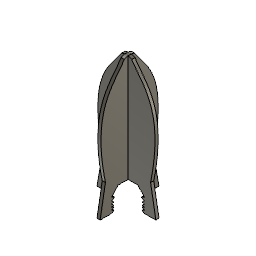
NYE-Rocket (Autodesk Fusion 360 design; units mm, degrees)
part number: 2025-12-20-13-37-46-259
Autodesk Fusion 360 part; units mm, degrees
sketch "Sketch1" plane through (0, 0, 0) normal (0, 1, 0) x (1, 0, 0)
  arc A0 (-14.7, 0) -> (-13.8108, -14.2595) centre (8.3307, -5.7213) ccw construction
  line L0 (0, 0) -> (0, -143.1953)
  line L1 (-11.7114, -15.7) -> (-12.05, -15.7) construction
  line L2 (-10.3, -17.45) -> (-10.3, -17.2374) construction
  arc A1 (-13.8108, -14.2595) -> (-11.7114, -15.7) centre (-11.7114, -13.45) ccw construction
  arc A2 (-10.3, -17.45) -> (-12.05, -15.7) centre (-12.05, -17.45) ccw construction
  arc A3 (-10.3, -17.2374) -> (-9.3791, -18.4433) centre (-9.05, -17.2374) ccw construction
  line L3 (11.7114, -15.7) -> (12.05, -15.7) construction
  arc A4 (11.7114, -15.7) -> (13.8108, -14.2595) centre (11.7114, -13.45) ccw construction
  arc A5 (13.8108, -14.2595) -> (14.7, 0) centre (-8.3307, -5.7213) ccw construction
  arc A6 (12.05, -15.7) -> (10.3, -17.45) centre (12.05, -17.45) ccw construction
  arc A7 (9.3791, -18.4433) -> (10.3, -17.2374) centre (9.05, -17.2374) ccw construction
  line L4 (10.3, -17.45) -> (10.3, -17.2374) construction
  arc A8 (0, -19.7) -> (9.3791, -18.4433) centre (0, 15.9286) ccw construction
  line L5 (-14.7, 0) -> (14.7, 0) construction
  line L6 (-27.5, 0) -> (-22.5628, -28)
  arc A9 (-5, -118.6603) -> (5, -118.6603) centre (0, -110) ccw
  line L7 (-22.5628, -28) -> (-35.5651, -92.1831) construction
  line L8 (-35.5651, -92.1831) -> (-14.6245, -102.766) construction
  line L9 (-14.6245, -102.766) -> (-5, -118.6603) construction
  spline S0 degree 3 poles (-22.5628, -28) (-35.5651, -92.1831) (-14.6245, -102.766) (-5, -118.6603) knots 0 0 0 0 1 1 1 1
  line L10 (-27.5, 0) -> (-16.6335, 0)
  line L11 (-16.6335, 0) -> (-14.2715, -1.5)
  line L12 (-14.2715, -1.5) -> (-16.6335, -2.7339)
  line L13 (-16.6335, -2.7339) -> (-14.6044, -4.2507)
  line L14 (-14.6044, -4.2507) -> (-16.6335, -5.1213)
  line L15 (-16.6335, -5.1213) -> (-14.65, -5.7122)
  line L16 (-14.65, -5.7122) -> (-16.6335, -7.5886)
  line L17 (-16.6335, -7.5886) -> (-14.5182, -8.2188)
  line L18 (-14.5182, -8.2188) -> (-16.6335, -10.2198)
  line L19 (-16.6335, -10.2198) -> (-13.8558, -11.8091)
  line L20 (-13.8558, -11.8091) -> (-16.6335, -13.4273)
  line L21 (-16.6335, -13.4273) -> (-10.5442, -19.9101)
  line L22 (-10.5442, -19.9101) -> (0, -19.9101)
  spline S1 degree 3 poles (22.5628, -28) (35.5651, -92.1831) (14.6245, -102.766) (5, -118.6603) knots 0 0 0 0 1 1 1 1
  line L23 (22.5628, -28) -> (35.5651, -92.1831) construction
  line L24 (35.5651, -92.1831) -> (14.6245, -102.766) construction
  line L25 (14.6245, -102.766) -> (5, -118.6603) construction
  line L26 (27.5, 0) -> (22.5628, -28)
  line L27 (27.5, 0) -> (16.6335, 0)
  line L28 (16.6335, -5.1213) -> (14.65, -5.7122)
  line L29 (14.65, -5.7122) -> (16.6335, -7.5886)
  line L30 (16.6335, -7.5886) -> (14.5182, -8.2188)
  line L31 (14.5182, -8.2188) -> (16.6335, -10.2198)
  line L32 (16.6335, -10.2198) -> (13.8558, -11.8091)
  line L33 (13.8558, -11.8091) -> (16.6335, -13.4273)
  line L34 (16.6335, -13.4273) -> (10.5442, -19.9101)
  line L35 (10.5442, -19.9101) -> (0, -19.9101)
  line L36 (14.6044, -4.2507) -> (16.6335, -5.1213)
  line L37 (16.6335, 0) -> (14.2715, -1.5)
  line L38 (14.2715, -1.5) -> (16.6335, -2.7339)
  line L39 (16.6335, -2.7339) -> (14.6044, -4.2507)
  line L40 (-1.575, -119.8752) -> (-1.575, -69.8752)
  line L41 (-1.575, -69.8752) -> (0, -69.8752)
  line L42 (1.575, -69.8752) -> (0, -69.8752)
  line L43 (1.575, -119.8752) -> (1.575, -69.8752)
  point P0 (-13.2, -15.7)
  point P1 (-10.3, -15.7)
  point P2 (10.3, -15.7)
  point P3 (13.2, -15.7)
  point P4 (-15.0215, -1.5)
  point P5 (-15.3544, -4.2507)
  point P6 (-15.4, -5.7122)
  point P7 (-15.2682, -8.2188)
  point P8 (-14.6058, -11.8091)
  dimension "d1" = 26.4
  dimension "d3" = 29.4
  dimension "d4" = 20.6
  dimension "d5" = 2.25
  dimension "d6" = 1.75
  dimension "d8" = 15.7
  dimension "d9" = 15.4
  dimension "d10" = 1.25
  dimension "d13" = 120
  dimension "d15" = 55
  dimension "d16" = 10
  dimension "d17" = 10
  dimension "d19" = 28
  dimension "d20" = 80
  dimension "d22" = 60
  dimension "d23" = 60
  dimension "d25" = 0.75
  dimension "d26" = 0.75
  dimension "d27" = 0.75
  dimension "d28" = 0.75
  dimension "d30" = 60
  dimension "d31" = 60
  dimension "d32" = 60
  dimension "d33" = 0.75
  dimension "d34" = 1.5
  dimension "d35" = 3.15
  dimension "d37" = 50
  constraint coincident L0.start origin
  constraint vertical L0
  constraint horizontal L1
  constraint perpendicular L1 L2
  constraint coincident P0 L1
  constraint coincident P0 A0
  constraint tangent A0 A1
  constraint tangent L1 A1
  constraint coincident P1 L1
  constraint coincident P1 L2
  constraint tangent L1 A2
  constraint tangent L2 A2
  constraint horizontal L0.start A0.start
  constraint tangent L2 A3
  constraint symmetric P0 L0 P3
  constraint symmetric A0.start L0 A5.end
  constraint symmetric A0 L0 A5
  constraint symmetric L0 P1 P2
  constraint symmetric L0 L1.start L3.start
  constraint symmetric L0 A0.end A4.end
  constraint symmetric L0 A1 A4
  constraint symmetric L0 L1.end L3.end
  constraint symmetric L0 L2.start A6.end
  constraint symmetric L0 A2 A6
  constraint symmetric L0 L2.end A7.end
  constraint symmetric L0 A3.end A7.start
  constraint symmetric L0 A3 A7
  constraint coincident A0.start L5.start
  constraint coincident A5.end L5.end
  constraint horizontal L0.start L6.start
  constraint symmetric L0 A9.start A9.end
  constraint parallel L5 L10
  constraint parallel L15 L17
  constraint coincident L0 L22.end
  constraint perpendicular L0 L22
  constraint coincident A0 P4
  constraint horizontal L11.end P4
  constraint coincident A0 P5
  constraint horizontal L13.end P5
  constraint coincident A0 P6
  constraint horizontal L15.end P6
  constraint coincident A0 P7
  constraint horizontal L17.end P7
  constraint coincident A0 P8
  constraint horizontal L19.end P8
  constraint vertical L18.end L20.end
  constraint vertical L16.end L18.end
  constraint vertical L14.end L16.end
  constraint vertical L12.end L14.end
  constraint vertical L10.end L12.end
  constraint symmetric L0 L6.start L26.start
  constraint symmetric L0 L6.end S1.start
  constraint symmetric L0 S0 S1
  constraint symmetric L0 L10.end L27.end
  constraint symmetric L0 L11.end L37.end
  constraint symmetric L0 L12.end L38.end
  constraint symmetric L0 L13.end L36.start
  constraint symmetric L0 L14.end L28.start
  constraint symmetric L0 L15.end L28.end
  constraint symmetric L0 L16.end L29.end
  constraint symmetric L0 L17.end L30.end
  constraint symmetric L0 L18.end L31.end
  constraint symmetric L0 L19.end L32.end
  constraint symmetric L0 L20.end L33.end
  constraint symmetric L0 L21.end L34.end
  constraint symmetric L0 L22.end L35.end
  constraint coincident A9 L40.start
  constraint vertical L40
  constraint perpendicular L40 L41
  constraint symmetric L0 L40.start L43.start
  constraint symmetric L0 L40.end L42.start
  constraint symmetric L0 L41.end L42.end
  measures "d5" radius of A1
  measures "d6" radius of A2
  measures "d8" vertical distance of A0.start L1.start
  measures "d9" distance of A0 L0
  measures "d10" radius of A3
  measures "d16" distance of A9.start A9.end
  measures "d17" radius of A9
  measures "d19" vertical distance of L6.start L6.end
  measures "d20" angle of L5 L6
  measures "d22" angle of L11 L12
  measures "d23" angle of L13 L14
  measures "d25" distance of L11.end P4
  measures "d26" distance of L13.end P5
  measures "d27" distance of L15.end P6
  measures "d28" distance of L17.end P7
  measures "d30" angle of L15 L16
  measures "d31" angle of L17 L18
  measures "d32" angle of L19 L20
  measures "d33" distance of L19.end P8
  measures "d34" distance of L10 L11.end
  measures "d37" distance of L40.start L40.end
sketch "Sketch3" plane through (0, 0, 0) normal (1, 0, 0) x (0, 1, 0)
  line L0 (1.575, -119.8752) -> (1.575, -69.8752)
  arc A0 (-10.3, -17.2374) -> (-9.3791, -18.4433) centre (-9.05, -17.2374) ccw construction
  line L1 (-16.6335, -5.1213) -> (-14.65, -5.7122)
  line L2 (-14.7, 0) -> (14.7, 0) construction
  line L3 (-16.6335, -2.7339) -> (-14.6044, -4.2507)
  line L4 (-10.3, -17.45) -> (-10.3, -17.2374) construction
  line L5 (1.575, -69.8752) -> (0, -69.8752)
  spline S0 degree 3 poles (-22.5628, -28) (-35.5651, -92.1831) (-14.6245, -102.766) (-5, -118.6603) knots 0 0 0 0 1 1 1 1
  line L6 (-22.5628, -28) -> (-35.5651, -92.1831) construction
  line L7 (-35.5651, -92.1831) -> (-14.6245, -102.766) construction
  line L8 (-14.6245, -102.766) -> (-5, -118.6603) construction
  line L9 (-10.5442, -19.9101) -> (0, -19.9101)
  line L10 (-16.6335, 0) -> (-14.2715, -1.5)
  line L11 (-27.5, 0) -> (-22.5628, -28)
  arc A1 (-14.7, 0) -> (-13.8108, -14.2595) centre (8.3307, -5.7213) ccw construction
  line L12 (27.5, 0) -> (22.5628, -28)
  arc A2 (-10.3, -17.45) -> (-12.05, -15.7) centre (-12.05, -17.45) ccw construction
  spline S1 degree 3 poles (22.5628, -28) (35.5651, -92.1831) (14.6245, -102.766) (5, -118.6603) knots 0 0 0 0 1 1 1 1
  line L13 (22.5628, -28) -> (35.5651, -92.1831) construction
  line L14 (35.5651, -92.1831) -> (14.6245, -102.766) construction
  line L15 (14.6245, -102.766) -> (5, -118.6603) construction
  line L16 (-1.575, -69.8752) -> (0, -69.8752)
  line L17 (-1.575, -119.8752) -> (-1.575, -69.8752)
  line L18 (16.6335, 0) -> (14.2715, -1.5)
  line L19 (14.6044, -4.2507) -> (16.6335, -5.1213)
  line L20 (14.2715, -1.5) -> (16.6335, -2.7339)
  line L21 (16.6335, -7.5886) -> (14.5182, -8.2188)
  line L22 (14.5182, -8.2188) -> (16.6335, -10.2198)
  line L23 (-16.6335, -7.5886) -> (-14.5182, -8.2188)
  line L24 (-14.5182, -8.2188) -> (-16.6335, -10.2198)
  line L25 (14.65, -5.7122) -> (16.6335, -7.5886)
  line L26 (-16.6335, -10.2198) -> (-13.8558, -11.8091)
  line L27 (-16.6335, -13.4273) -> (-10.5442, -19.9101)
  line L28 (-14.2715, -1.5) -> (-16.6335, -2.7339)
  line L29 (-11.7114, -15.7) -> (-12.05, -15.7) construction
  arc A3 (-13.8108, -14.2595) -> (-11.7114, -15.7) centre (-11.7114, -13.45) ccw construction
  line L30 (-27.5, 0) -> (-16.6335, 0)
  arc A4 (9.3791, -18.4433) -> (10.3, -17.2374) centre (9.05, -17.2374) ccw construction
  line L31 (-14.6044, -4.2507) -> (-16.6335, -5.1213)
  line L32 (10.5442, -19.9101) -> (0, -19.9101)
  line L33 (27.5, 0) -> (16.6335, 0)
  line L34 (16.6335, -5.1213) -> (14.65, -5.7122)
  line L35 (16.6335, -13.4273) -> (10.5442, -19.9101)
  arc A5 (13.8108, -14.2595) -> (14.7, 0) centre (-8.3307, -5.7213) ccw construction
  line L36 (11.7114, -15.7) -> (12.05, -15.7) construction
  arc A6 (0, -19.7) -> (9.3791, -18.4433) centre (0, 15.9286) ccw construction
  line L37 (13.8558, -11.8091) -> (16.6335, -13.4273)
  arc A7 (11.7114, -15.7) -> (13.8108, -14.2595) centre (11.7114, -13.45) ccw construction
  line L38 (16.6335, -2.7339) -> (14.6044, -4.2507)
  line L39 (10.3, -17.45) -> (10.3, -17.2374) construction
  line L40 (16.6335, -10.2198) -> (13.8558, -11.8091)
  arc A8 (12.05, -15.7) -> (10.3, -17.45) centre (12.05, -17.45) ccw construction
  arc A9 (-5, -118.6603) -> (5, -118.6603) centre (0, -110) ccw
  line L41 (-13.8558, -11.8091) -> (-16.6335, -13.4273)
  line L42 (-14.65, -5.7122) -> (-16.6335, -7.5886)
  line L43 (1.75, 0) -> (22.5, 0)
  line L44 (10.3, 17.45) -> (10.3, 17.2374) construction
  line L45 (11.7114, 15.7) -> (12.05, 15.7) construction
  line L46 (14.65, 5.7122) -> (16.6335, 7.5886)
  arc A10 (10.3, 17.2374) -> (9.3791, 18.4433) centre (9.05, 17.2374) ccw construction
  line L47 (16.6335, 5.1213) -> (14.65, 5.7122)
  line L48 (10.5442, 19.9101) -> (0, 19.9101)
  line L49 (27.5, 0) -> (22.5628, 28)
  line L50 (14.6044, 4.2507) -> (16.6335, 5.1213)
  line L51 (-27.5, 0) -> (-22.5628, 28)
  arc A11 (9.3791, 18.4433) -> (0, 19.7) centre (0, -15.9286) ccw construction
  line L52 (16.6335, 10.2198) -> (13.8558, 11.8091)
  line L53 (14.2715, 1.5) -> (16.6335, 2.7339)
  line L54 (-10.5442, 19.9101) -> (0, 19.9101)
  line L55 (13.8558, 11.8091) -> (16.6335, 13.4273)
  line L56 (-14.7, 0) -> (14.7, 0) construction
  spline S2 degree 3 poles (22.5628, 28) (35.5651, 92.1831) (14.6245, 102.766) (5, 118.6603) knots 0 0 0 0 1 1 1 1
  line L57 (22.5628, 28) -> (35.5651, 92.1831) construction
  line L58 (35.5651, 92.1831) -> (14.6245, 102.766) construction
  line L59 (14.6245, 102.766) -> (5, 118.6603) construction
  arc A12 (14.7, 0) -> (13.8108, 14.2595) centre (-8.3307, 5.7213) ccw construction
  spline S3 degree 3 poles (-22.5628, 28) (-35.5651, 92.1831) (-14.6245, 102.766) (-5, 118.6603) knots 0 0 0 0 1 1 1 1
  line L60 (-22.5628, 28) -> (-35.5651, 92.1831) construction
  line L61 (-35.5651, 92.1831) -> (-14.6245, 102.766) construction
  line L62 (-14.6245, 102.766) -> (-5, 118.6603) construction
  arc A13 (10.3, 17.45) -> (12.05, 15.7) centre (12.05, 17.45) ccw construction
  line L63 (-1.575, 69.8752) -> (0, 69.8752)
  line L64 (-14.6044, 4.2507) -> (-16.6335, 5.1213)
  line L65 (16.6335, 13.4273) -> (10.5442, 19.9101)
  line L66 (1.575, 69.8752) -> (0, 69.8752)
  line L67 (-14.65, 5.7122) -> (-16.6335, 7.5886)
  line L68 (14.5182, 8.2188) -> (16.6335, 10.2198)
  arc A14 (-13.8108, 14.2595) -> (-14.7, 0) centre (8.3307, 5.7213) ccw construction
  arc A15 (5, 118.6603) -> (-5, 118.6603) centre (0, 110) ccw
  line L69 (-16.6335, 10.2198) -> (-13.8558, 11.8091)
  line L70 (27.5, 0) -> (16.6335, 0)
  line L71 (-14.5182, 8.2188) -> (-16.6335, 10.2198)
  arc A16 (13.8108, 14.2595) -> (11.7114, 15.7) centre (11.7114, 13.45) ccw construction
  line L72 (16.6335, 0) -> (14.2715, 1.5)
  line L73 (-16.6335, 7.5886) -> (-14.5182, 8.2188)
  line L74 (-16.6335, 5.1213) -> (-14.65, 5.7122)
  line L75 (-16.6335, 0) -> (-14.2715, 1.5)
  line L76 (16.6335, 7.5886) -> (14.5182, 8.2188)
  line L77 (-16.6335, 13.4273) -> (-10.5442, 19.9101)
  arc A17 (-9.3791, 18.4433) -> (-10.3, 17.2374) centre (-9.05, 17.2374) ccw construction
  arc A18 (-12.05, 15.7) -> (-10.3, 17.45) centre (-12.05, 17.45) ccw construction
  line L78 (-11.7114, 15.7) -> (-12.05, 15.7) construction
  line L79 (16.6335, 2.7339) -> (14.6044, 4.2507)
  line L80 (-13.8558, 11.8091) -> (-16.6335, 13.4273)
  line L81 (-14.2715, 1.5) -> (-16.6335, 2.7339)
  line L82 (-16.6335, 2.7339) -> (-14.6044, 4.2507)
  line L83 (-10.3, 17.45) -> (-10.3, 17.2374) construction
  line L84 (-27.5, 0) -> (-16.6335, 0)
  arc A19 (-11.7114, 15.7) -> (-13.8108, 14.2595) centre (-11.7114, 13.45) ccw construction
  line L85 (-1.575, 69.8752) -> (-1.575, 19.9101)
  line L86 (0, 0) -> (0, 28)
  line L87 (1.575, 69.8752) -> (1.575, 19.9101)
  point P0 (-13.2, -15.7)
  point P1 (10.3, -15.7)
  point P2 (13.2, -15.7)
  point P3 (-15.3544, -4.2507)
  point P4 (-15.2682, -8.2188)
  point P5 (-14.6058, -11.8091)
  point P6 (-15.4, -5.7122)
  point P7 (-15.0215, -1.5)
  point P8 (-10.3, -15.7)
  point P9 (-14.6058, 11.8091)
  point P10 (-15.2682, 8.2188)
  point P11 (10.3, 15.7)
  point P12 (-15.0215, 1.5)
  point P13 (-13.2, 15.7)
  point P14 (-15.3544, 4.2507)
  point P15 (13.2, 15.7)
  point P16 (-10.3, 15.7)
  point P17 (-15.4, 5.7122)
  dimension "d68" = 2.25
  dimension "d69" = 1.75
  dimension "d70" = 15.7
  dimension "d71" = 1.25
  dimension "d72" = 120
  dimension "d73" = 10
  dimension "d74" = 10
  dimension "d75" = 28
  dimension "d76" = 80
  dimension "d77" = 60
  dimension "d78" = 60
  dimension "d79" = 0.75
  dimension "d80" = 0.75
  dimension "d81" = 0.75
  dimension "d82" = 0.75
  dimension "d83" = 60
  dimension "d84" = 60
  dimension "d85" = 60
  dimension "d86" = 0.75
  dimension "d87" = 1.5
  dimension "d88" = 50
  dimension "d89" = 3.15
  constraint coincident L86.start origin
  constraint horizontal L29
  constraint perpendicular L4 L29
  constraint coincident P0 L29
  constraint coincident P0 A1
  constraint tangent A1 A3
  constraint tangent L29 A3
  constraint coincident P8 L29
  constraint coincident P8 L4
  constraint tangent A2 L29
  constraint tangent L4 A2
  constraint horizontal L86.start L2.start
  constraint tangent A0 L4
  constraint coincident L2.start A1.start
  constraint coincident L2.end A5.end
  constraint horizontal L11.start L86.start
  constraint parallel L2 L30
  constraint parallel L1 L23
  constraint coincident P7 A1
  constraint horizontal P7 L10.end
  constraint coincident P3 A1
  constraint horizontal P3 L3.end
  constraint coincident P6 A1
  constraint horizontal L1.end P6
  constraint coincident P4 A1
  constraint horizontal L23.end P4
  constraint coincident P5 A1
  constraint horizontal L26.end P5
  constraint vertical L27.start L24.end
  constraint vertical L24.end L23.start
  constraint vertical L1.start L23.start
  constraint vertical L1.start L3.start
  constraint vertical L3.start L10.start
  constraint coincident L17.start A9
  constraint vertical L17
  constraint perpendicular L16 L17
  constraint symmetric L86.start L43 origin
  constraint symmetric A4.end L43 L44.end
  constraint symmetric A1.end L43 A14.start
  constraint symmetric L11.start L43 L30.start
  constraint symmetric S0.start L43 L51.end
  constraint symmetric L9.end L43 L48.end
  constraint symmetric P0 L43 P13
  constraint symmetric S0.end L43 S3.end
  constraint symmetric L29.start L43 L78.start
  constraint symmetric L23.end L43 L71.start
  constraint symmetric L4.start L43 A18.end
  constraint symmetric A2.end L43 A18.start
  constraint symmetric L2.start L43 A1.start
  constraint symmetric L36.start L43 L45.start
  constraint symmetric A6.start L43 A11.end
  constraint symmetric S1.end L43 S2.end
  constraint symmetric L36.end L43 L45.end
  constraint symmetric P1 L43 P11
  constraint symmetric L2.end L43 A5.end
  constraint symmetric P2 L43 P15
  constraint symmetric A5.start L43 A12.end
  constraint symmetric A4.start L43 A10.end
  constraint symmetric L39.start L43 L44.start
  constraint symmetric P3 L43 P14
  constraint symmetric L1.start L43 L64.end
  constraint symmetric L26.end L43 L69.end
  constraint symmetric L27.start L43 L77.start
  constraint symmetric L3.end L43 L64.start
  constraint symmetric L3.start L43 L81.end
  constraint symmetric L0.end L43 L66.start
  constraint symmetric L9.start L43 L54.start
  constraint symmetric P4 L43 P10
  constraint symmetric P5 L43 P9
  constraint symmetric L1.end L43 L67.start
  constraint symmetric L5.end L43 L63.end
  constraint symmetric L32.start L43 L48.start
  constraint symmetric L12.start L43 L33.start
  constraint symmetric L18.start L43 L33.end
  constraint symmetric L21.start L43 L46.end
  constraint symmetric L21.end L43 L68.start
  constraint symmetric L20.end L43 L53.end
  constraint symmetric L37.start L43 L52.end
  constraint symmetric L35.start L43 L55.end
  constraint symmetric L19.start L43 L50.start
  constraint symmetric L18.end L43 L53.start
  constraint symmetric L25.start L43 L46.start
  constraint symmetric L19.end L43 L47.start
  constraint symmetric L22.end L43 L52.start
  constraint symmetric L16.start L43 L63.start
  constraint symmetric L12.end L43 L49.end
  constraint symmetric P6 L43 P17
  constraint symmetric P7 L43 P12
  constraint symmetric A0.end L43 A17.start
  constraint symmetric A0.start L43 A17.end
  constraint symmetric P8 L43 P16
  constraint symmetric L10.end L43 L75.end
  constraint symmetric L24.end L43 L69.start
  constraint symmetric L23.start L43 L67.end
  constraint symmetric L10.start L43 L30.end
  constraint symmetric A0 L43 A17
  constraint symmetric S0 L43 S3
  constraint symmetric A1 L43 A14
  constraint symmetric A2 L43 A18
  constraint symmetric S1 L43 S2
  constraint symmetric A3 L43 A19
  constraint symmetric A4 L43 A10
  constraint symmetric A5 L43 A12
  constraint symmetric A6 L43 A11
  constraint symmetric A7 L43 A16
  constraint symmetric A8 L43 A13
  constraint symmetric A9 L43 A15
  constraint coincident L54 L85.end
  constraint perpendicular L54 L85
  constraint symmetric L63.start L86 L66.start
  constraint symmetric L85.end L86 L87.end
  measures "d68" radius of A3
  measures "d69" radius of A2
  measures "d70" vertical distance of L29.start L2.start
  measures "d71" radius of A0
  measures "d73" distance of S0.end S1.end
  measures "d74" radius of A9
  measures "d75" distance of L11.start S0.start
  measures "d76" angle of L2 L11
  measures "d77" angle of L10 L28
  measures "d78" angle of L3 L31
  measures "d79" distance of P7 L10.end
  measures "d80" distance of P3 L3.end
  measures "d81" distance of L1.end P6
  measures "d82" distance of L23.end P4
  measures "d83" angle of L1 L42
  measures "d84" angle of L23 L24
  measures "d85" angle of L26 L41
  measures "d86" distance of L26.end P5
  measures "d87" distance of L10.end L30
  measures "d88" distance of L17.start L16.start
  measures "d89" distance of L85 L87
extrude "Extrude1" add sketch "Sketch1" along normal mid plane 3 contours L0 A9 S1 L26 L27 L28 L29 L30 L31 L32 L33 L34 L35 L36 L37 L38 L39 L42 L43 | L0 L6 A9 S0 L10 L11 L12 L13 L14 L15 L16 L17 L18 L19 L20 L21 L22 L40 L41
extrude "Extrude2" add sketch "Sketch3" along normal mid plane 3 contours L30 L33 L43 L46 L47 L48 L49 L50 L51 L52 L53 L54 L55 S2 S3 L63 L64 L65 L66 L67 L68 A15 L69 L70 L71 L72 L73 L74 L75 L76 L77 L79 L80 L81 L82 L84 L85 L87
equation "d9 = ( 30.8 / 2 ) * 1 mm"
equation "total_height = 120 mm"
equation "d13 = total_height"
equation "base_width = 55 mm" comment "Standing Fin Width"
equation "d15 = base_width"
equation "d17 = nose_radius"
equation "nose_radius = 10 mm" comment "Rocket Tip Radius"
equation "d22 = teeth_angle"
equation "d23 = teeth_angle"
equation "teeth_grip_depth = 0.75 mm" comment "How far the gripping teeth shall bite into the kork"
equation "d25 = teeth_grip_depth"
equation "d26 = teeth_grip_depth"
equation "d27 = teeth_grip_depth"
equation "d28 = teeth_grip_depth"
equation "teeth_angle = 60 deg" comment "How sharp the gripping teeth shall be"
equation "d30 = teeth_angle"
equation "d31 = teeth_angle"
equation "d32 = teeth_angle"
equation "d33 = teeth_grip_depth"
equation "d35 = material_thickness + pressfit_tolerance"
equation "material_thickness = 3 mm" comment "How thick the manufacturing material of both rocket sides is"
equation "d37 = ( 100 / 2 ) * 1 mm"
equation "d65 = material_thickness"
equation "pressfit_tolerance = 0.15 mm" comment "Tolerance that is given once for the intersecting rocket bodies. Depends on manufacturing technique."
equation "d72 = total_height"
equation "d74 = nose_radius"
equation "d77 = teeth_angle"
equation "d78 = teeth_angle"
equation "d79 = teeth_grip_depth"
equation "d80 = teeth_grip_depth"
equation "d81 = teeth_grip_depth"
equation "d82 = teeth_grip_depth"
equation "d83 = teeth_angle"
equation "d84 = teeth_angle"
equation "d85 = teeth_angle"
equation "d86 = teeth_grip_depth"
equation "d88 = ( 100 / 2 ) * 1 mm"
equation "d89 = material_thickness + pressfit_tolerance"
equation "d90 = material_thickness"
